Autodesk Inventor part; units mm, degrees
(part 2 of 2)
sketch "Sketch28" plane through (2.5, 0, 0) normal (1, 0, 0) x (0, 0, -1)
  line L0 (82, 17.8) -> (82, 5) projected
  line L1 (66, 17.8) -> (82, 17.8) projected
  line L2 (66, 5) -> (66, 17.8) projected
  line L3 (82, 5) -> (66, 5) projected
  line L4 (67.0532, 35.5) -> (67.0532, 21.8) projected
  line L5 (71.0532, 21.8) -> (71.0532, 35.5) projected
  line L6 (67.0532, 21.8) -> (63.0532, 21.8) projected
  line L7 (63.0532, 21.8) -> (63.0532, 35.5) projected
  line L8 (63.0532, 35.5) -> (67.0532, 35.5) projected
  line L9 (71.0532, 35.5) -> (75.0532, 35.5) projected
  line L10 (75.0532, 35.5) -> (75.0532, 21.8) projected
  line L11 (75.0532, 21.8) -> (71.0532, 21.8) projected
  line L12 (83.0532, 21.8) -> (79.0532, 21.8) projected
  line L13 (79.0532, 21.8) -> (79.0532, 35.5) projected
  line L14 (83.0532, 35.5) -> (83.0532, 21.8) projected
  line L15 (79.0532, 35.5) -> (83.0532, 35.5) projected
  line L16 (59.0532, 5.5) -> (55.0532, 5.5) projected
  line L17 (59.0532, 35.5) -> (59.0532, 5.5) projected
  line L18 (55.0532, 5.5) -> (55.0532, 35.5) projected
  line L19 (55.0532, 35.5) -> (59.0532, 35.5) projected
  line L20 (47.0532, 5.5) -> (47.0532, 35.5) projected
  line L21 (51.0532, 35.5) -> (51.0532, 5.5) projected
  line L22 (51.0532, 5.5) -> (47.0532, 5.5) projected
  line L23 (47.0532, 35.5) -> (51.0532, 35.5) projected
  line L24 (39.0532, 35.5) -> (43.0532, 35.5) projected
  line L25 (43.0532, 5.5) -> (39.0532, 5.5) projected
  line L26 (39.0532, 5.5) -> (39.0532, 35.5) projected
  line L27 (43.0532, 35.5) -> (43.0532, 5.5) projected
  point P0 (0, 0)
extrude "Extrusion27" add sketch "Sketch28" against normal up to surface (5 mm away) contours L0 L3 L2 L1 | L4 L6 L7 L8 | L5 L9 L10 L11 | L12 L13 L15 L14 | L16 L18 L19 L17 | L20 L23 L21 L22
sketch "Sketch29" plane through (2.5, 0, 0) normal (1, 0, 0) x (0, 0, -1)
  line L0 (15.0532, 35.5) -> (19.0532, 35.5) projected
  line L1 (19.0532, 35.5) -> (19.0532, 5.5) projected
  line L2 (19.0532, 5.5) -> (15.0532, 5.5) projected
  line L3 (15.0532, 5.5) -> (15.0532, 35.5) projected
  line L4 (31.0532, 35.5) -> (35.0532, 35.5) projected
  line L5 (35.0532, 35.5) -> (35.0532, 5.5) projected
  line L6 (35.0532, 5.5) -> (31.0532, 5.5) projected
  line L7 (31.0532, 5.5) -> (31.0532, 35.5) projected
  line L8 (23.0532, 35.5) -> (27.0532, 35.5) projected
  line L9 (27.0532, 35.5) -> (27.0532, 5.5) projected
  line L10 (27.0532, 5.5) -> (23.0532, 5.5) projected
  line L11 (23.0532, 5.5) -> (23.0532, 35.5) projected
  line L12 (39.0532, 35.5) -> (43.0532, 35.5) projected
  line L13 (43.0532, 35.5) -> (43.0532, 5.5) projected
  line L14 (43.0532, 5.5) -> (39.0532, 5.5) projected
  line L15 (39.0532, 5.5) -> (39.0532, 35.5) projected
  line L16 (87.0532, 35.5) -> (91.0532, 35.5) projected
  line L17 (91.0532, 35.5) -> (91.0532, 5.5) projected
  line L18 (91.0532, 5.5) -> (87.0532, 5.5) projected
  line L19 (87.0532, 5.5) -> (87.0532, 35.5) projected
  line L20 (95.0532, 35.5) -> (99.0532, 35.5) projected
  line L21 (99.0532, 35.5) -> (99.0532, 5.5) projected
  line L22 (99.0532, 5.5) -> (95.0532, 5.5) projected
  line L23 (95.0532, 5.5) -> (95.0532, 35.5) projected
  circle A0 centre (-30, 10) radius 2.6 projected
  circle A1 centre (-10, 10) radius 2.6 projected
  circle A2 centre (-10, 30) radius 2.6 projected
  circle A3 centre (-30, 30) radius 2.6 projected
  line L24 (112.7, 40) -> (-40, 40) projected
  line L25 (-40, 40) -> (-40, 0) projected
  line L26 (-40, 0) -> (124.7, 0) projected
  line L27 (124.7, 0) -> (124.7, 30.6) projected
  line L28 (124.7, 30.6) -> (112.7, 30.6) projected
  line L29 (112.7, 30.6) -> (112.7, 40) projected
  line L30 (43.0532, 20) -> (58.0532, 20)
  line L31 (58.0532, 20) -> (58.0532, 5)
  line L32 (58.0532, 5) -> (43.0532, 5)
  line L33 (43.0532, 5) -> (43.0532, 20)
  point P0 (0, 0)
  dimension "d199" = 0
  dimension "d200" = 15
  dimension "d201" = 15
  dimension "d202" = 5
  constraints: 8 end point, 2 parallel, 1 horizontal, 1 perpendicular
  measures "d199" distance between parallel lines of L13 L33
  measures "d200" distance of L30.start L30.end
  measures "d201" distance of L30.end L31.end
  measures "d202" distance between parallel lines of L26 L32
extrude "Extrusion28" cut sketch "Sketch29" against normal blind 10 contours L30 L31 L32 L33 L13
sketch "Sketch30" plane through (2.5, 0, 0) normal (1, 0, 0) x (0, 0, -1)
  line L0 (112.7, 40) -> (-40, 40) projected
  line L1 (-40, 40) -> (-40, 0) projected
  line L2 (-40, 0) -> (124.7, 0) projected
  line L3 (124.7, 0) -> (124.7, 30.6) projected
  line L4 (124.7, 30.6) -> (112.7, 30.6) projected
  line L5 (112.7, 30.6) -> (112.7, 40) projected
  circle A0 centre (-30, 30) radius 2.6 projected
  circle A1 centre (-10, 30) radius 2.6 projected
  circle A2 centre (-10, 10) radius 2.6 projected
  circle A3 centre (-30, 10) radius 2.6 projected
  line L6 (95.0532, 35.5) -> (99.0532, 35.5) projected
  line L7 (99.0532, 35.5) -> (99.0532, 5.5) projected
  line L8 (99.0532, 5.5) -> (95.0532, 5.5) projected
  line L9 (95.0532, 5.5) -> (95.0532, 35.5) projected
  line L10 (87.0532, 35.5) -> (91.0532, 35.5) projected
  line L11 (91.0532, 35.5) -> (91.0532, 5.5) projected
  line L12 (91.0532, 5.5) -> (87.0532, 5.5) projected
  line L13 (87.0532, 5.5) -> (87.0532, 35.5) projected
  line L14 (43.0532, 20) -> (58.0532, 20) projected
  line L15 (58.0532, 20) -> (58.0532, 5) projected
  line L16 (58.0532, 5) -> (43.0532, 5) projected
  line L17 (43.0532, 5) -> (43.0532, 5.5) projected
  line L18 (43.0532, 5.5) -> (39.0532, 5.5) projected
  line L19 (39.0532, 5.5) -> (39.0532, 35.5) projected
  line L20 (39.0532, 35.5) -> (43.0532, 35.5) projected
  line L21 (43.0532, 35.5) -> (43.0532, 20) projected
  line L22 (23.0532, 35.5) -> (27.0532, 35.5) projected
  line L23 (27.0532, 35.5) -> (27.0532, 5.5) projected
  line L24 (27.0532, 5.5) -> (23.0532, 5.5) projected
  line L25 (23.0532, 5.5) -> (23.0532, 35.5) projected
  line L26 (31.0532, 35.5) -> (35.0532, 35.5) projected
  line L27 (35.0532, 35.5) -> (35.0532, 5.5) projected
  line L28 (35.0532, 5.5) -> (31.0532, 5.5) projected
  line L29 (31.0532, 5.5) -> (31.0532, 35.5) projected
  line L30 (15.0532, 35.5) -> (19.0532, 35.5) projected
  line L31 (19.0532, 35.5) -> (19.0532, 5.5) projected
  line L32 (19.0532, 5.5) -> (15.0532, 5.5) projected
  line L33 (15.0532, 5.5) -> (15.0532, 35.5) projected
  line L34 (39.0532, 35.5) -> (43.0532, 35.5)
  line L35 (43.0532, 35.5) -> (43.0532, 5.5)
  line L36 (43.0532, 5.5) -> (39.0532, 5.5)
  line L37 (39.0532, 5.5) -> (39.0532, 35.5)
  point P0 (0, 0)
  constraints: 8 end point, 2 parallel, 1 horizontal, 1 perpendicular
extrude "Extrusion29" add sketch "Sketch30" against normal up to surface (5 mm away) contours L35 L18 L19 L20 L21
sketch "Sketch31" plane through (2.5, 0, 0) normal (1, 0, 0) x (0, 0, -1)
  line L0 (112.7, 40) -> (-40, 40) projected
  line L1 (-40, 40) -> (-40, 0) projected
  line L2 (-40, 0) -> (124.7, 0) projected
  line L3 (124.7, 0) -> (124.7, 30.6) projected
  line L4 (124.7, 30.6) -> (112.7, 30.6) projected
  line L5 (112.7, 30.6) -> (112.7, 40) projected
  circle A0 centre (-30, 30) radius 2.6 projected
  circle A1 centre (-10, 30) radius 2.6 projected
  circle A2 centre (-10, 10) radius 2.6 projected
  circle A3 centre (-30, 10) radius 2.6 projected
  line L6 (95.0532, 35.5) -> (99.0532, 35.5) projected
  line L7 (99.0532, 35.5) -> (99.0532, 5.5) projected
  line L8 (99.0532, 5.5) -> (95.0532, 5.5) projected
  line L9 (95.0532, 5.5) -> (95.0532, 35.5) projected
  line L10 (87.0532, 35.5) -> (91.0532, 35.5) projected
  line L11 (91.0532, 35.5) -> (91.0532, 5.5) projected
  line L12 (91.0532, 5.5) -> (87.0532, 5.5) projected
  line L13 (87.0532, 5.5) -> (87.0532, 35.5) projected
  line L14 (43.0532, 20) -> (58.0532, 20) projected
  line L15 (58.0532, 20) -> (58.0532, 5) projected
  line L16 (58.0532, 5) -> (43.0532, 5) projected
  line L17 (43.0532, 5) -> (43.0532, 20) projected
  line L18 (23.0532, 35.5) -> (27.0532, 35.5) projected
  line L19 (27.0532, 35.5) -> (27.0532, 5.5) projected
  line L20 (27.0532, 5.5) -> (23.0532, 5.5) projected
  line L21 (23.0532, 5.5) -> (23.0532, 35.5) projected
  line L22 (31.0532, 35.5) -> (35.0532, 35.5) projected
  line L23 (35.0532, 35.5) -> (35.0532, 5.5) projected
  line L24 (35.0532, 5.5) -> (31.0532, 5.5) projected
  line L25 (31.0532, 5.5) -> (31.0532, 35.5) projected
  line L26 (15.0532, 35.5) -> (19.0532, 35.5) projected
  line L27 (19.0532, 35.5) -> (19.0532, 5.5) projected
  line L28 (19.0532, 5.5) -> (15.0532, 5.5) projected
  line L29 (15.0532, 5.5) -> (15.0532, 35.5) projected
  line L30 (83.0532, 35.5) -> (79.0532, 35.5) projected
  line L31 (83.0532, 5.5) -> (79.0532, 5.5)
  line L32 (79.0532, 5.5) -> (79.0532, 35.5)
  line L33 (79.0532, 35.5) -> (83.0532, 35.5)
  line L34 (83.0532, 35.5) -> (83.0532, 5.5)
  line L35 (75.0532, 35.5) -> (71.0532, 35.5)
  line L36 (71.0532, 35.5) -> (71.0532, 5.5)
  line L37 (71.0532, 5.5) -> (75.0532, 5.5)
  line L38 (75.0532, 5.5) -> (75.0532, 35.5)
  line L39 (67.0532, 35.5) -> (63.0532, 35.5)
  line L40 (63.0532, 35.5) -> (63.0532, 5.5)
  line L41 (63.0532, 5.5) -> (67.0532, 5.5)
  line L42 (67.0532, 5.5) -> (67.0532, 35.5)
  line L43 (59.0532, 35.5) -> (55.0532, 35.5)
  line L44 (55.0532, 35.5) -> (55.0532, 24)
  line L45 (55.0532, 24) -> (59.0532, 24)
  line L46 (59.0532, 24) -> (59.0532, 35.5)
  line L47 (51.0532, 24) -> (47.0532, 24)
  line L48 (47.0532, 24) -> (47.0532, 35.5)
  line L49 (47.0532, 35.5) -> (51.0532, 35.5)
  line L50 (51.0532, 35.5) -> (51.0532, 24)
  line L51 (43.0532, 24) -> (39.0532, 24)
  line L52 (39.0532, 24) -> (39.0532, 35.5)
  line L53 (39.0532, 35.5) -> (43.0532, 35.5)
  line L54 (43.0532, 35.5) -> (43.0532, 24)
  point P0 (0, 0)
  dimension "d207" = 4
  dimension "d208" = 4
  dimension "d209" = 4
  dimension "d210" = 4
  dimension "d211" = 4
  dimension "d212" = 4
  dimension "d213" = 4
  dimension "d214" = 4
  dimension "d215" = 0
  dimension "d216" = 4
  dimension "d217" = 4
  dimension "d218" = 4
  dimension "d219" = 4
  dimension "d220" = 4
  constraints: 48 end point, 12 parallel, 7 point on line, 6 horizontal, 6 perpendicular
  measures "d207" distance of L32.end L33.end
  measures "d208" distance of L37.end L36.end
  measures "d209" distance of L41.end L40.end
  measures "d210" distance between parallel lines of L13 L34
  measures "d211" distance between parallel lines of L38 L32
  measures "d212" distance between parallel lines of L36 L42
  measures "d213" distance of L45.end L44.end
  measures "d214" distance between parallel lines of L14 L45
  measures "d215" distance between parallel lines of L39 L43
  measures "d216" distance of L48.end L49.end
  measures "d217" distance of L52.end L53.end
  measures "d218" distance between parallel lines of L50 L44
  measures "d219" distance between parallel lines of L54 L48
  measures "d220" distance between parallel lines of L40 L46
extrude "Extrusion30" cut sketch "Sketch31" against normal blind 10 contours L34 L31 L32 L30 | L38 L37 L36 L35 | L42 L41 L40 L39 | L46 L45 L44 L43 | L47 L48 L49 L50 | L51 L52 L53 L54
sketch "Sketch33" plane through (0, 2, 0) normal (0, 1, 0) x (1, 0, 0)
  line L0 (-11, 124.7) -> (-11, 107.2) projected
  line L1 (-11, 124.7) -> (-113, 124.7) projected
  line L2 (-113, 107.2) -> (-113, 124.7) projected
  arc A0 (-116, 104.2) -> (-113, 107.2) centre (-116, 107.2) ccw projected
  line L3 (-121.5, 104.2) -> (-116, 104.2) projected
  line L4 (-121.5, 11.25) -> (-121.5, 104.2) projected
  line L5 (-116, 11.25) -> (-121.5, 11.25) projected
  arc A1 (-113, 8.25) -> (-116, 11.25) centre (-116, 8.25) ccw projected
  line L6 (-113, 2.5) -> (-113, 8.25) projected
  line L7 (-11, 2.5) -> (-113, 2.5) projected
  line L8 (-11, 8.25) -> (-11, 2.5) projected
  arc A2 (-8, 11.25) -> (-11, 8.25) centre (-8, 8.25) ccw projected
  line L9 (-2.5, 11.25) -> (-8, 11.25) projected
  line L10 (-2.5, 104.2) -> (-2.5, 11.25) projected
  line L11 (-8, 104.2) -> (-2.5, 104.2) projected
  arc A3 (-11, 107.2) -> (-8, 104.2) centre (-8, 107.2) ccw projected
  circle A4 centre (-27.9, 26.9) radius 1.35
  circle A5 centre (-27.9, 26.9) radius 2.5
  circle A6 centre (-103.9, 26.9) radius 2.5
  circle A7 centre (-103.9, 26.9) radius 1.35
  line L12 (-2.5, 112.7) -> (-2.5, 2.5) projected
  line L13 (-2.5, 2.5) -> (-121.5, 2.5) projected
  line L14 (-121.5, 112.7) -> (-121.5, 2.5) projected
  line L15 (-121.5, 112.7) -> (-124, 112.7) projected
  line L16 (-124, 0) -> (-124, 112.7) projected
  line L17 (0, 0) -> (-124, 0) projected
  line L18 (0, 0) -> (0, -40) projected
  line L19 (0, -40) -> (2.5, -40) projected
  line L20 (2.5, 112.7) -> (2.5, -40) projected
  line L21 (2.5, 112.7) -> (-2.5, 112.7) projected
  point P0 (0, 0)
  dimension "d234" = 2.7
  dimension "d235" = 5
  dimension "d236" = 5
  dimension "d237" = 2.7
  dimension "d238" = 30.4
  dimension "d239" = 76
  dimension "d240" = 97.8
  dimension "d241" = 97.8
  constraints: 4 centre point, 2 coincident
  measures "d234" diameter of A4
  measures "d235" diameter of A5
  measures "d236" diameter of A6
  measures "d237" diameter of A7
  measures "d238" distance from line of L20 A4.centre
  measures "d239" distance of A7.centre A4.centre
  measures "d240" distance from line of L1 A6.centre
  measures "d241" distance from line of L1 A5.centre
extrude "Extrusion32" add sketch "Sketch33" along normal blind 3 contours A5 | A6
sketch "Sketch34" plane through (0, 2, 0) normal (0, 1, 0) x (1, 0, 0)
  circle A0 centre (-27.9, 26.9) radius 2.5 projected
  circle A1 centre (-103.9, 26.9) radius 2.5 projected
  line L0 (-11, 124.7) -> (-11, 107.2) projected
  line L1 (-11, 124.7) -> (-113, 124.7) projected
  line L2 (-113, 107.2) -> (-113, 124.7) projected
  arc A2 (-116, 104.2) -> (-113, 107.2) centre (-116, 107.2) ccw projected
  line L3 (-121.5, 104.2) -> (-116, 104.2) projected
  line L4 (-121.5, 11.25) -> (-121.5, 104.2) projected
  line L5 (-116, 11.25) -> (-121.5, 11.25) projected
  arc A3 (-113, 8.25) -> (-116, 11.25) centre (-116, 8.25) ccw projected
  line L6 (-113, 2.5) -> (-113, 8.25) projected
  line L7 (-11, 2.5) -> (-113, 2.5) projected
  line L8 (-11, 8.25) -> (-11, 2.5) projected
  arc A4 (-8, 11.25) -> (-11, 8.25) centre (-8, 8.25) ccw projected
  line L9 (-2.5, 11.25) -> (-8, 11.25) projected
  line L10 (-2.5, 104.2) -> (-2.5, 11.25) projected
  line L11 (-8, 104.2) -> (-2.5, 104.2) projected
  arc A5 (-11, 107.2) -> (-8, 104.2) centre (-8, 107.2) ccw projected
  circle A6 centre (-103.9, 26.9) radius 1.35 projected
  circle A7 centre (-27.9, 26.9) radius 1.35 projected
  point P0 (0, 0)
extrude "Extrusion33" cut sketch "Sketch34" against normal blind 1 contours A6 | A7
fillet "Fillet4" radius 3 2 edges at (-106.4, 2, -26.9) (-30.4, 2, -26.9)
ref_plane "Work Plane3" through (-2.5, 0, 0) normal (-1, 0, 0) x (0, 0, 1)
sketch "Sketch35" plane through (-2.5, 0, 0) normal (-1, 0, 0) x (0, 0, 1)
  line L0 (0, 0) -> (0, 40) projected
  line L1 (40, 0) -> (0, 0) projected
  line L2 (40, 40) -> (40, 0) projected
  line L3 (0, 40) -> (40, 40) projected
  circle A0 centre (30, 10) radius 2.6 projected
  circle A1 centre (10, 10) radius 2.6 projected
  circle A2 centre (10, 30) radius 2.6 projected
  circle A3 centre (30, 30) radius 2.6 projected
  line L4 (40.1751, 40.1639) -> (-141.3847, 40.1639)
  line L5 (-141.3847, 40.1639) -> (-141.3847, -6.9272)
  line L6 (-141.3847, -6.9272) -> (40.1751, -6.9272)
  line L7 (40.1751, -6.9272) -> (40.1751, 40.1639)
  constraints: 8 end point, 2 parallel, 1 horizontal, 1 perpendicular
extrude "Extrusion34" cut sketch "Sketch35" along normal through all contours L7 L6 L5 L4
sketch "Sketch36" plane through (-1.5, 30.6, -126.2) normal (0, 1, 0) x (1, 0, 0)
  line L0 (-1, 2) -> (-1, 0) projected
  line L1 (0, 0) -> (-1, 0) projected
  line L2 (0, 1) -> (0, 0) projected
  line L3 (-1, 2) -> (0, 1) projected
  point P0 (1.5, -126.2)
extrude "Extrusion35" cut sketch "Sketch36" against normal through all
sketch "Sketch37" plane through (2.5, 0, 0) normal (1, 0, 0) x (0, 0, -1)
  line L0 (71.0532, 5.5) -> (71.0532, 35.5) projected
  line L1 (71.0532, 35.5) -> (75.0532, 35.5) projected
  line L2 (75.0532, 35.5) -> (75.0532, 5.5) projected
  line L3 (75.0532, 5.5) -> (71.0532, 5.5) projected
  line L4 (43.0532, 35.5) -> (43.0532, 24) projected
  line L5 (43.0532, 24) -> (39.0532, 24) projected
  line L6 (39.0532, 24) -> (39.0532, 35.5) projected
  line L7 (39.0532, 35.5) -> (43.0532, 35.5) projected
  line L8 (55.0532, 24) -> (55.0532, 35.5) projected
  line L9 (55.0532, 35.5) -> (59.0532, 35.5) projected
  line L10 (59.0532, 35.5) -> (59.0532, 24) projected
  line L11 (59.0532, 24) -> (55.0532, 24) projected
  line L12 (51.0532, 35.5) -> (51.0532, 24) projected
  line L13 (51.0532, 24) -> (47.0532, 24) projected
  line L14 (47.0532, 24) -> (47.0532, 35.5) projected
  line L15 (47.0532, 35.5) -> (51.0532, 35.5) projected
  line L16 (83.0532, 35.5) -> (83.0532, 5.5) projected
  line L17 (83.0532, 5.5) -> (79.0532, 5.5) projected
  line L18 (79.0532, 5.5) -> (79.0532, 35.5) projected
  line L19 (79.0532, 35.5) -> (83.0532, 35.5) projected
  line L20 (63.0532, 5.5) -> (63.0532, 35.5) projected
  line L21 (63.0532, 35.5) -> (67.0532, 35.5) projected
  line L22 (67.0532, 35.5) -> (67.0532, 5.5) projected
  line L23 (67.0532, 5.5) -> (63.0532, 5.5) projected
  line L24 (112.7, 40) -> (-40, 40) projected
  line L25 (-40, 40) -> (-40, 0) projected
  line L26 (-40, 0) -> (124.7, 0) projected
  line L27 (124.7, 0) -> (124.7, 30.6) projected
  line L28 (124.7, 30.6) -> (112.7, 30.6) projected
  line L29 (112.7, 30.6) -> (112.7, 40) projected
  circle A0 centre (-30, 30) radius 2.6 projected
  circle A1 centre (-10, 30) radius 2.6 projected
  circle A2 centre (-10, 10) radius 2.6 projected
  circle A3 centre (-30, 10) radius 2.6 projected
  line L30 (95.0532, 35.5) -> (99.0532, 35.5) projected
  line L31 (99.0532, 35.5) -> (99.0532, 5.5) projected
  line L32 (99.0532, 5.5) -> (95.0532, 5.5) projected
  line L33 (95.0532, 5.5) -> (95.0532, 35.5) projected
  line L34 (87.0532, 35.5) -> (91.0532, 35.5) projected
  line L35 (91.0532, 35.5) -> (91.0532, 5.5) projected
  line L36 (91.0532, 5.5) -> (87.0532, 5.5) projected
  line L37 (87.0532, 5.5) -> (87.0532, 35.5) projected
  line L38 (43.0532, 20) -> (58.0532, 20) projected
  line L39 (58.0532, 20) -> (58.0532, 5) projected
  line L40 (58.0532, 5) -> (43.0532, 5) projected
  line L41 (43.0532, 5) -> (43.0532, 20) projected
  line L42 (23.0532, 35.5) -> (27.0532, 35.5) projected
  line L43 (27.0532, 35.5) -> (27.0532, 5.5) projected
  line L44 (27.0532, 5.5) -> (23.0532, 5.5) projected
  line L45 (23.0532, 5.5) -> (23.0532, 35.5) projected
  line L46 (31.0532, 35.5) -> (35.0532, 35.5) projected
  line L47 (35.0532, 35.5) -> (35.0532, 5.5) projected
  line L48 (35.0532, 5.5) -> (31.0532, 5.5) projected
  line L49 (31.0532, 5.5) -> (31.0532, 35.5) projected
  line L50 (15.0532, 35.5) -> (19.0532, 35.5) projected
  line L51 (19.0532, 35.5) -> (19.0532, 5.5) projected
  line L52 (19.0532, 5.5) -> (15.0532, 5.5) projected
  line L53 (15.0532, 5.5) -> (15.0532, 35.5) projected
  line L54 (124.7, 30.6) -> (112.7, 30.6) projected
  line L55 (112.7, 30.6) -> (124.7, 30.6)
  line L56 (124.7, 30.6) -> (124.7, 0)
  line L57 (124.7, 0) -> (112.7, 0)
  line L58 (112.7, 0) -> (112.7, 30.6)
  point P0 (0, 0)
  constraints: 8 end point, 2 parallel, 1 horizontal, 1 perpendicular
extrude "Extrusion36" cut sketch "Sketch37" against normal blind 10 contours L28 L27 L26 L58
sketch "Sketch38" plane through (2.5, 0, 0) normal (1, 0, 0) x (0, 0, -1)
  line L0 (15.0532, 35.5) -> (19.0532, 35.5) projected
  line L1 (19.0532, 35.5) -> (19.0532, 5.5) projected
  line L2 (19.0532, 5.5) -> (15.0532, 5.5) projected
  line L3 (15.0532, 5.5) -> (15.0532, 35.5) projected
  line L4 (31.0532, 35.5) -> (35.0532, 35.5) projected
  line L5 (35.0532, 35.5) -> (35.0532, 5.5) projected
  line L6 (35.0532, 5.5) -> (31.0532, 5.5) projected
  line L7 (31.0532, 5.5) -> (31.0532, 35.5) projected
  line L8 (23.0532, 35.5) -> (27.0532, 35.5) projected
  line L9 (27.0532, 35.5) -> (27.0532, 5.5) projected
  line L10 (27.0532, 5.5) -> (23.0532, 5.5) projected
  line L11 (23.0532, 5.5) -> (23.0532, 35.5) projected
  line L12 (43.0532, 20) -> (58.0532, 20) projected
  line L13 (58.0532, 20) -> (58.0532, 5) projected
  line L14 (58.0532, 5) -> (43.0532, 5) projected
  line L15 (43.0532, 5) -> (43.0532, 20) projected
  line L16 (87.0532, 35.5) -> (91.0532, 35.5) projected
  line L17 (91.0532, 35.5) -> (91.0532, 5.5) projected
  line L18 (91.0532, 5.5) -> (87.0532, 5.5) projected
  line L19 (87.0532, 5.5) -> (87.0532, 35.5) projected
  line L20 (95.0532, 35.5) -> (99.0532, 35.5) projected
  line L21 (99.0532, 35.5) -> (99.0532, 5.5) projected
  line L22 (99.0532, 5.5) -> (95.0532, 5.5) projected
  line L23 (95.0532, 5.5) -> (95.0532, 35.5) projected
  circle A0 centre (-30, 10) radius 2.6 projected
  circle A1 centre (-10, 10) radius 2.6 projected
  circle A2 centre (-10, 30) radius 2.6 projected
  circle A3 centre (-30, 30) radius 2.6 projected
  line L24 (112.7, 0) -> (112.7, 40) projected
  line L25 (112.7, 40) -> (-40, 40) projected
  line L26 (-40, 40) -> (-40, 0) projected
  line L27 (-40, 0) -> (112.7, 0) projected
  line L28 (63.0532, 5.5) -> (63.0532, 35.5) projected
  line L29 (63.0532, 35.5) -> (67.0532, 35.5) projected
  line L30 (67.0532, 35.5) -> (67.0532, 5.5) projected
  line L31 (67.0532, 5.5) -> (63.0532, 5.5) projected
  line L32 (83.0532, 35.5) -> (83.0532, 5.5) projected
  line L33 (83.0532, 5.5) -> (79.0532, 5.5) projected
  line L34 (79.0532, 5.5) -> (79.0532, 35.5) projected
  line L35 (79.0532, 35.5) -> (83.0532, 35.5) projected
  line L36 (51.0532, 35.5) -> (51.0532, 24) projected
  line L37 (51.0532, 24) -> (47.0532, 24) projected
  line L38 (47.0532, 24) -> (47.0532, 35.5) projected
  line L39 (47.0532, 35.5) -> (51.0532, 35.5) projected
  line L40 (55.0532, 24) -> (55.0532, 35.5) projected
  line L41 (55.0532, 35.5) -> (59.0532, 35.5) projected
  line L42 (59.0532, 35.5) -> (59.0532, 24) projected
  line L43 (59.0532, 24) -> (55.0532, 24) projected
  line L44 (43.0532, 35.5) -> (43.0532, 24) projected
  line L45 (43.0532, 24) -> (39.0532, 24) projected
  line L46 (39.0532, 24) -> (39.0532, 35.5) projected
  line L47 (39.0532, 35.5) -> (43.0532, 35.5) projected
  line L48 (71.0532, 5.5) -> (71.0532, 35.5) projected
  line L49 (71.0532, 35.5) -> (75.0532, 35.5) projected
  line L50 (75.0532, 35.5) -> (75.0532, 5.5) projected
  line L51 (75.0532, 5.5) -> (71.0532, 5.5) projected
  circle A4 centre (6.875, 27.5) radius 1.5
  circle A5 centre (6.875, 10) radius 1.5
  circle A6 centre (108.45, 27.5) radius 1.5
  circle A7 centre (108.45, 10) radius 1.5
  point P0 (0, 0)
  dimension "d254" = 3
  dimension "d255" = 3
  dimension "d256" = 3
  dimension "d257" = 3
  dimension "d258" = 10
  dimension "d259" = 10
  dimension "d260" = 12.5
  dimension "d261" = 12.5
  dimension "d264" = 4.25
  dimension "d265" = 4.25
  dimension "d266" = 101.575
  dimension "d267" = 101.575
  constraints: 4 centre point
  measures "d254" diameter of A4
  measures "d255" diameter of A5
  measures "d256" diameter of A6
  measures "d257" diameter of A7
  measures "d258" distance from line of L27 A5.centre
  measures "d259" distance from line of L27 A7.centre
  measures "d260" distance from line of L25 A6.centre
  measures "d261" distance from line of L25 A4.centre
  measures "d264" distance from line of L24 A6.centre
  measures "d265" distance from line of L24 A7.centre
  measures "d266" distance of A6.centre A4.centre
  measures "d267" distance of A7.centre A5.centre
extrude "Extrusion37" cut sketch "Sketch38" against normal blind 10 contours A4 | A5 | A6 | A7
body "Solid1"
